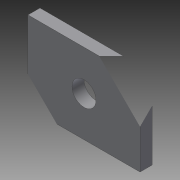
# Autodesk Inventor part: arm_plate
Saved by Autodesk Inventor 2015 (Build 190159000, 159)
## iProperties
Created: 2015-06-21
Part Number: arm_plate
Material: Generic
Document SubType Name: Modeling
Designer: Master
Density: 1 g/cm^3
Appearance: Default
Author: Master
Autodesk Inventor part; units mm, degrees
ref_plane "YZ Plane" through (0, 0, 0) normal (1, 0, 0) x (0, 1, 0)
ref_plane "XZ Plane" through (0, 0, 0) normal (0, 1, 0) x (-1, 0, 0)
ref_plane "XY Plane" through (0, 0, 0) normal (0, 0, 1) x (1, 0, 0)
sketch "Sketch1" plane through (0, 0, 0) normal (0, 0, 1) x (1, 0, 0)
  line L0 (-14, -0.25) -> (0, -0.25) projected
  line L1 (0, -0.25) -> (0, 0) projected
  line L2 (0, 0) -> (0, 10) projected
  line L3 (0, 10) -> (0, 10.25) projected
  line L4 (0, 10.25) -> (-14, 10.25) projected
  line L5 (-14, 10.25) -> (-14, -0.25) projected
  circle A0 centre (-7, 5) radius 1.5 projected
  line L6 (0, 0) -> (-14, 0)
  line L7 (-14, 0) -> (-14, 10)
  line L8 (-14, 10) -> (0, 10)
  line L9 (0, 10) -> (0, 0)
  dimension "d0" = 0.25
  dimension "d1" = 0.25
  constraints: 8 end point, 2 point on line
  measures "d0" distance between parallel lines of L0 L6
  measures "d1" distance between parallel lines of L8 L4
extrude "Extrusion1" add sketch "Sketch1" along normal blind 1.5 contours L5 L8 L2 L6
body "Solid1"
